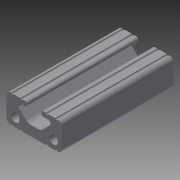
# Autodesk Inventor part: 1050-2-CL
Saved by Autodesk Inventor 2014 SP2 (Build 180246200, 246)
## iProperties
Created: 2019-08-30
Part Number: 1050-2-CL
Material: Generic
Catalog Web Link: www.cadenas.de
Description: 1050, 1050-Black-FB-T-Slotted Profile - 10 Series
Vendor: 8020
Document SubType Name: Modeling
Designer: psadmin
Manufacturer: 8020
Mass: 10.4706 g
Surface Area: 69.095 cm^2
Volume: 10.4706 cm^3
Density: 1 g/cm^3
Appearance: PSOLRGB-191-191-191
Category: PARTsolutions
Company: 8020
Title: 1050-2
Author: Cadenas PARTsolutions
Comments: T-Slotted Profile - 10 Series
PSOL_IDENT_0: {$CADENAS_DATA\23d-libs\8020\inch\profiles\10_series\1050.prj},180 {VTYP=3D},{NB=1050-2-CL},{LINA=10
PSOL_IDENT_1: 50-2},{NN=1050, 1050-Black-FB},{DATE=04.12.2018 10:30:19},{GEOMDATE=09.02.2018 14:28:57},{VERSION=},
PSOL_IDENT_2: {LINEID=10},{WBVAR=FINISH,LS,L},{WBNUMERIC=L}  {NB=1050-2-CL},{LINA=1050-2},{KT=DUMMY},{PN=1050-2},{
PSOL_IDENT_3: SERIES=1050},{MAT=6105-T5 Aluminum},{FINISH=CA},{LS=-CL},{L=2.000},{LALG=[1:145/0.005]},{W=.3679},{M
PSOL_IDENT_4: IX=.0074},{MIY=.0323},{EA=.3161},{CLR=.75,.75,.75}
NN: 1050, 1050-Black-FB
NT: T-Slotted Profile - 10 Series
NB: 1050-2-CL
NBSYN: $PN.$LS.
LINA: 1050-2
PN: 1050-2
SERIES: 1050
MAT: 6105-T5 Aluminum
FINISH: Clear Anodize
LS: Custom Length
L: 2
W: .3679
MIX: .0074
MIY: .0323
EA: .3161
SUPPLIER: 8020
ARTICLENO: 1050-2-CL
BOMINFO: 1050-2
CREATOR: CADENAS GmbH
Autodesk Inventor part; units mm, degrees
ref_plane "YZ Plane" through (0, 0, 0) normal (1, 0, 0) x (0, 1, 0)
ref_plane "XZ Plane" through (0, 0, 0) normal (0, 1, 0) x (-1, 0, 0)
ref_plane "XY Plane" through (0, 0, 0) normal (0, 0, 1) x (1, 0, 0)
sketch "Sketch_1" plane through (0, 0, 0) normal (0, 0, 1) x (1, 0, 0)
  arc A0 (-12.7, 2.1082) -> (-10.5791, 0) centre (-10.5918, 2.1082) ccw
  arc A1 (-9.5504, 0) -> (-10.5791, 0) centre (-10.0648, -0.0064) ccw
  line L0 (-9.5504, 0) -> (-6.3246, 0)
  arc A2 (-5.3086, 0) -> (-6.3246, 0) centre (-5.8166, 0) ccw
  line L1 (-5.3086, 0) -> (5.3086, 0)
  arc A3 (6.3246, 0) -> (5.3086, 0) centre (5.8166, 0) ccw
  line L2 (6.3246, 0) -> (9.5504, 0)
  arc A4 (10.5791, 0) -> (9.5504, 0) centre (10.0648, -0.0064) ccw
  arc A5 (10.5791, 0) -> (12.7, 2.1082) centre (10.5918, 2.1082) ccw
  line L3 (12.7, 2.1082) -> (12.7, 10.5918)
  arc A6 (12.7, 10.5918) -> (10.5791, 12.7) centre (10.5918, 10.5918) ccw
  arc A7 (9.5504, 12.7) -> (10.5791, 12.7) centre (10.0648, 12.7064) ccw
  line L4 (9.5504, 12.7) -> (6.3246, 12.7)
  arc A8 (5.3086, 12.7) -> (6.3246, 12.7) centre (5.8166, 12.7) ccw
  line L5 (5.3086, 12.7) -> (4.3023, 12.7)
  arc A9 (4.3023, 12.7) -> (4.3023, 10.4902) centre (4.3023, 11.5951) ccw
  line L6 (4.3023, 10.4902) -> (6.488, 10.4902)
  arc A10 (7.2064, 8.7558) -> (6.488, 10.4902) centre (6.488, 9.4742) ccw
  line L7 (7.2064, 8.7558) -> (3.8763, 5.4257)
  arc A11 (1.6313, 4.4958) -> (3.8763, 5.4257) centre (1.6313, 7.6708) ccw
  line L8 (1.6313, 4.4958) -> (-1.6313, 4.4958)
  arc A12 (-3.8763, 5.4257) -> (-1.6313, 4.4958) centre (-1.6313, 7.6708) ccw
  line L9 (-3.8763, 5.4257) -> (-7.2064, 8.7558)
  arc A13 (-6.488, 10.4902) -> (-7.2064, 8.7558) centre (-6.488, 9.4742) ccw
  line L10 (-6.488, 10.4902) -> (-4.3023, 10.4902)
  arc A14 (-4.3023, 10.4902) -> (-4.3023, 12.7) centre (-4.3023, 11.5951) ccw
  line L11 (-4.3023, 12.7) -> (-5.3086, 12.7)
  arc A15 (-6.3246, 12.7) -> (-5.3086, 12.7) centre (-5.8166, 12.7) ccw
  line L12 (-6.3246, 12.7) -> (-9.5504, 12.7)
  arc A16 (-10.5791, 12.7) -> (-9.5504, 12.7) centre (-10.0648, 12.7064) ccw
  arc A17 (-10.5791, 12.7) -> (-12.7, 10.5918) centre (-10.5918, 10.5918) ccw
  line L13 (-12.7, 10.5918) -> (-12.7, 2.1082)
  circle A18 centre (8.7312, 3.9624) radius 2.032
  circle A19 centre (-8.7312, 3.9624) radius 2.032
  constraints: 36 point on circle, 28 end point, 20 centre point
extrude "Extrusion1" add sketch "Sketch_1" against normal blind 50.8
body "Solid1"
